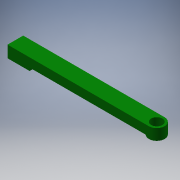
# Autodesk Inventor part: barraConector
Saved by Autodesk Inventor 2016 (Build 200138000, 138)
## iProperties
Created: 2020-03-18
Part Number: barraConector
Material: Genérico
Document SubType Name: Modeling
Designer: Andres Gomez
Density: 1 g/cm^3
Appearance: Verde oscuro
Author: Andres Gomez
Autodesk Inventor part; units mm, degrees
ref_plane "YZ Plane" through (0, 0, 0) normal (1, 0, 0) x (0, 1, 0)
ref_plane "XZ Plane" through (0, 0, 0) normal (0, 1, 0) x (-1, 0, 0)
ref_plane "XY Plane" through (0, 0, 0) normal (0, 0, 1) x (1, 0, 0)
sketch "Boceto1" plane through (0, 0, 0) normal (0, 0, 1) x (1, 0, 0)
  circle A0 centre (0, 0) radius 7.65
  circle A1 centre (0, 0) radius 10.65
  dimension "d0" = 15.3
  dimension "d1" = 21.3
  constraints: 2 centre point, 2 coincident
  measures "d0" diameter of A0
  measures "d1" diameter of A1
extrude "Extrusión1" add sketch "Boceto1" against normal blind 15
sketch "Boceto4" plane through (0, 0, 0) normal (0, 0, 1) x (1, 0, 0)
  circle A0 centre (0, 0) radius 10.65 projected
  line L0 (0, -10.65) -> (-192, -10.65)
  line L1 (0, -10.65) -> (192, -10.65) construction
  line L2 (0, 10.65) -> (-192, 10.65)
  line L3 (-192, 10.65) -> (-192, -10.65)
  dimension "d4" = 192
  dimension "d5" = 180
  constraints: 8 end point, 3 horizontal, 2 point on circle, 1 collinear, 1 perpendicular, 1 tangent
  measures "d4" distance of L0.start L0.end
  measures "d5" angle of L0 L1
extrude "Extrusión2" add sketch "Boceto4" against normal blind 12 contours A0 L0 L3 L2
sketch "Boceto17" plane through (0, 0, -12) normal (0, 0, -1) x (-1, 0, 0)
  line L0 (192, -10.65) -> (192, 10.65) projected
  line L1 (0, -10.65) -> (192, -10.65) projected
  line L2 (192, 10.65) -> (162, 10.65)
  line L3 (162, 10.65) -> (162, -10.65)
  line L4 (162, -10.65) -> (192, -10.65)
  line L5 (192, -10.65) -> (192, 10.65)
  point P0 (0, 0)
  dimension "d75" = 30
  constraints: 8 end point, 2 parallel, 1 horizontal, 1 perpendicular, 1 point on line
  measures "d75" distance of L4.end L3.end
extrude "Extrusión14" add sketch "Boceto17" along normal blind 4
sketch "Boceto18" plane through (0, 0, -16) normal (0, 0, -1) x (-1, 0, 0)
  circle A0 centre (184.7091, -0.6121) radius 5
  point P0 (0, 0)
  dimension "d78" = 10
  constraints: 1 centre point
  measures "d78" diameter of A0
extrude "Extrusión15" cut sketch "Boceto18" against normal blind 16
sketch "Boceto19" plane through (0, 0, -16) normal (0, 0, -1) x (-1, 0, 0)
  circle A0 centre (184.8056, -0.7065) radius 4.9956
  circle A1 centre (184.8056, -0.7065) radius 6
  point P0 (0, 0)
  dimension "d81" = 12
  constraints: 2 centre point, 1 coincident
  measures "d81" diameter of A1
extrude "Extrusión16" add sketch "Boceto19" along normal blind 1
fillet "Empalme10" radius 0.5 1 edges at (-178.8056, -0.7065, -17)
fillet "Empalme11" radius 8 2 edges at (-192, 10.65, -8) (-192, -10.65, -8)
sketch "Boceto20" plane through (0, 0, 0) normal (0, 0, 1) x (1, 0, 0)
  circle A0 centre (-184.7809, -0.6444) radius 5
  circle A1 centre (-184.7809, -0.6444) radius 6
  point P0 (0, 0)
  dimension "d86" = 10
  dimension "d87" = 12
  constraints: 2 centre point, 1 coincident
  measures "d86" diameter of A0
  measures "d87" diameter of A1
extrude "Extrusión17" add sketch "Boceto20" along normal blind 1
fillet "Empalme12" radius 0.5 1 edges at (-190.7809, -0.6444, 1)
fillet "Empalme13" radius 2 1 edges at (-162, 0, -16)
fillet "Empalme14" radius 1 1 edges at (-10.65, 0, -15)
sketch "Boceto21" plane through (0, 0, -12) normal (0, 0, -1) x (-1, 0, 0)
  line L0 (155.2699, -6.6555) -> (22.8192, -6.6555)
  line L1 (22.8192, -6.6555) -> (22.8192, -15.3654)
  line L2 (22.8192, -15.3654) -> (155.2699, -15.3654)
  line L3 (155.2699, -15.3654) -> (155.2699, -6.6555)
  line L4 (155.2699, 5.3804) -> (22.8192, 5.3804)
  line L5 (22.8192, 5.3804) -> (22.8192, 12.897)
  line L6 (22.8192, 12.897) -> (155.2699, 12.897)
  line L7 (155.2699, 12.897) -> (155.2699, 5.3804)
  point P0 (0, 0)
  constraints: 16 end point, 4 parallel, 2 horizontal, 2 perpendicular
extrude "Extrusión18" cut sketch "Boceto21" against normal blind 24
fillet "Empalme15" radius 2 4 edges at (-22.8192, 10.65, -6) (-22.8192, -10.65, -6) (-155.2699, 10.65, -6) (-155.2699, -10.65, -6)
fillet "Empalme16" radius 2 4 edges at (-89.0446, 5.3804, -12) (-89.0446, -6.6555, -12) (-89.0446, 5.3804, 0) (-89.0446, -6.6555, 0)
